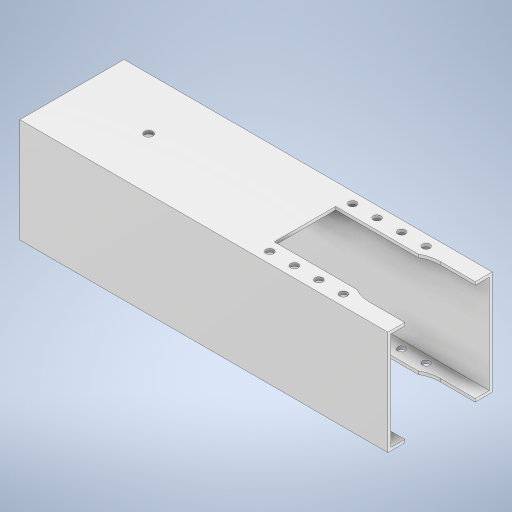
# Autodesk Inventor part: Eslabon_L
Saved by Autodesk Inventor 2024 (Build 280153000, 153)
## iProperties
Created: 2023-05-25
Part Number: Eslabon_L
Material: Plástico ABS
Document SubType Name: Modeling
Designer: epm01
Density: 1.06 g/cm^3
Appearance: Suave - Blanco
Author: epm01
Autodesk Inventor part; units mm, degrees
ref_plane "YZ Plane" through (0, 0, 0) normal (1, 0, 0) x (0, 1, 0)
ref_plane "XZ Plane" through (0, 0, 0) normal (0, 1, 0) x (-1, 0, 0)
ref_plane "XY Plane" through (0, 0, 0) normal (0, 0, 1) x (1, 0, 0)
sketch "Boceto1" plane through (0, 0, 0) normal (1, 0, 0) x (0, 1, 0)
  line L0 (-16, 16) -> (16, 16)
  line L1 (16, 16) -> (16, -16)
  line L2 (16, -16) -> (-16, -16)
  line L3 (-16, -16) -> (-16, 16)
  line L4 (-16, 16) -> (16, -16) construction
  line L5 (16, 16) -> (-16, -16) construction
  line L6 (17, 17) -> (-17, 17)
  line L7 (-17, 17) -> (-17, -17)
  line L8 (-17, -17) -> (17, -17)
  line L9 (17, -17) -> (17, 17)
  line L10 (17, 17) -> (-17, -17) construction
  line L11 (-17, 17) -> (17, -17) construction
  point P0 (0, 0)
  dimension "d0" = 32
  dimension "d1" = 32
  dimension "d2" = 34
  dimension "d3" = 34
  constraints: 24 end point, 4 midpoint, 4 parallel, 2 horizontal, 2 perpendicular, 1 point on line
  measures "d0" distance of L0.start L0.end
  measures "d1" distance of L0.end L1.end
  measures "d2" distance of L6.start L6.end
  measures "d3" distance of L8.end L6.start
extrude "Extrusión1" add sketch "Boceto1" along normal blind 100
sketch "Boceto5" plane through (0, 17, 17) normal (0, 1, 0) x (1, 0, 0)
  line L0 (100, 1) -> (100, 33) projected
  line L1 (100, 17) -> (88.5, 17) construction
  line L2 (88.5, 17) -> (82, 17) construction
  line L3 (82, 17) -> (82, 30.5) construction
  circle A0 centre (82, 30.5) radius 1.25
  circle A1 centre (74, 30.5) radius 1.25
  line L4 (80.5, 17) -> (74, 17) construction
  circle A2 centre (66, 30.5) radius 1.25
  line L5 (72.5, 17) -> (66, 17) construction
  circle A3 centre (58, 30.5) radius 1.25
  line L6 (64.5, 17) -> (58, 17) construction
  circle A4 centre (82, 3.5) radius 1.25
  line L7 (88.5, -10) -> (82, -10) construction
  circle A5 centre (74, 3.5) radius 1.25
  line L8 (80.5, -10) -> (74, -10) construction
  circle A6 centre (66, 3.5) radius 1.25
  line L9 (72.5, -10) -> (66, -10) construction
  circle A7 centre (58, 3.5) radius 1.25
  line L10 (64.5, -10) -> (58, -10) construction
  circle A8 centre (88.5, 17) radius 11.5
  point P0 (0, 17)
  dimension "d26" = 11.5
  dimension "d27" = 6.5
  dimension "d28" = 13.5
  dimension "d29" = 2.5
  dimension "d32" = 8
  dimension "d35" = 27
  dimension "d38" = 23
  constraints: 20 end point, 9 centre point, 2 coincident, 2 horizontal, 2 vertical, 1 collinear, 1 midpoint, 1 point on line, 34 other
  measures "d26" distance of L1.start L1.end
  measures "d27" distance of L1.end L2.end
  measures "d28" distance of L2.end L3.end
  measures "d29" diameter of A0
  measures "d32" distance of A0.centre A1.centre
  measures "d35" distance of A0.centre A4.centre
  measures "d38" diameter of A8
extrude "Extrusión4" cut sketch "Boceto5" against normal through all
sketch "Boceto6" plane through (0, 17, 17) normal (0, 1, 0) x (1, 0, 0)
  line L0 (100, 17) -> (100, 34) projected
  line L1 (100, 17) -> (56, 17) construction
  line L2 (0, 0) -> (100, 0) projected
  line L3 (56, 0) -> (56, 7) construction
  line L4 (56, 34) -> (56, 27) construction
  line L5 (56, 27) -> (56, 7)
  line L6 (56, 7) -> (83.498, 7)
  line L7 (56, 0) -> (56, 7) construction
  line L8 (56, 27) -> (83.498, 27)
  line L9 (83.498, 27) -> (83.498, 7)
  point P0 (0, 17)
  dimension "d41" = 44
  dimension "d42" = 7
  constraints: 16 end point, 5 symmetric about line, 2 horizontal, 2 vertical, 1 collinear, 1 point on line
  measures "d41" distance of L0.start L1.end
  measures "d42" distance of L3.start L3.end
extrude "Extrusión5" cut sketch "Boceto6" against normal through all
sketch "Boceto7" plane through (0, 17, 17) normal (0, 1, 0) x (1, 0, 0)
  arc A0 (100, 17) -> (82.8211, 27) centre (88.5, 17) ccw projected
  line L0 (88.5, 17) -> (88.5, 28.5)
  line L1 (88.5, 28.5) -> (103.9894, 28.5)
  line L2 (88.5, 17) -> (100, 17) construction
  line L3 (88.5, 17) -> (88.5, 5.5)
  line L4 (88.5, 5.5) -> (103.9894, 5.5)
  line L5 (103.9894, 28.5) -> (103.9894, 5.5)
  point P0 (0, 17)
  constraints: 12 end point, 2 horizontal, 2 symmetric about line, 2 vertical, 1 point on circle, 1 tangent
extrude "Extrusión6" cut sketch "Boceto7" against normal through all
sketch "Boceto8" plane through (0, 17, 17) normal (0, 1, 0) x (1, 0, 0)
  line L0 (0, 17) -> (5, 17)
  dimension "d47" = 5
  constraints: 2 end point, 1 horizontal
  measures "d47" distance of L0.start L0.end
hole "Agujero1" at (5, 17, 0) direction (0, -1, 0) diameter 2.75 end through all
sketch "Boceto9" plane through (0, 0, 0) normal (-1, 0, 0) x (0, 0, 1)
  line L0 (-11.5, 16) -> (-16, 16) projected
  line L1 (11.5, -16) -> (16, -16) projected
  line L2 (-16, 16) -> (16, 16)
  line L3 (16, 16) -> (16, -16)
  line L4 (16, -16) -> (-16, -16)
  line L5 (-16, -16) -> (-16, 16)
  line L6 (-17, 17) -> (17, 17) projected
  line L7 (17, 17) -> (17, -17) projected
  line L8 (-17, 17) -> (17, 17)
  line L9 (17, 17) -> (17, -17)
  line L10 (17, -17) -> (-17, -17)
  line L11 (-17, -17) -> (-17, 17)
  point P0 (0, 0)
  constraints: 16 end point, 4 parallel, 2 horizontal, 2 perpendicular
extrude "Extrusión7" add sketch "Boceto9" along normal blind 20
